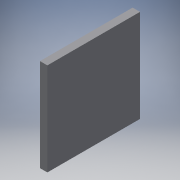
# Autodesk Inventor part: XCarve
Saved by Autodesk Inventor 2017 (Build 210142000, 142)
## iProperties
Created: 2017-06-27
Part Number: XCarve
Material: Generic
Document SubType Name: Modeling
Designer: sensor
Density: 1 g/cm^3
Appearance: Default
Author: sensor
Autodesk Inventor part; units mm, degrees
ref_plane "YZ Plane" through (0, 0, 0) normal (1, 0, 0) x (0, 1, 0)
ref_plane "XZ Plane" through (0, 0, 0) normal (0, 1, 0) x (-1, 0, 0)
ref_plane "XY Plane" through (0, 0, 0) normal (0, 0, 1) x (1, 0, 0)
sketch "Sketch1" plane through (0, 0, 0) normal (1, 0, 0) x (0, 1, 0)
  line L0 (445.5446, 19.802) -> (-554.4554, 19.802)
  line L1 (-554.4554, 19.802) -> (-554.4554, -980.198)
  line L2 (-554.4554, -980.198) -> (445.5446, -980.198)
  line L3 (445.5446, -980.198) -> (445.5446, 19.802)
  point P0 (0, 0)
  dimension "d0" = 1000
  dimension "d1" = 1000
  constraints: 8 end point, 2 parallel, 1 horizontal, 1 perpendicular
  measures "d0" distance of L2.end L0.start
  measures "d1" distance of L1.end L2.end
extrude "Extrusion1" add sketch "Sketch1" along normal blind 80
body "Solid1"
